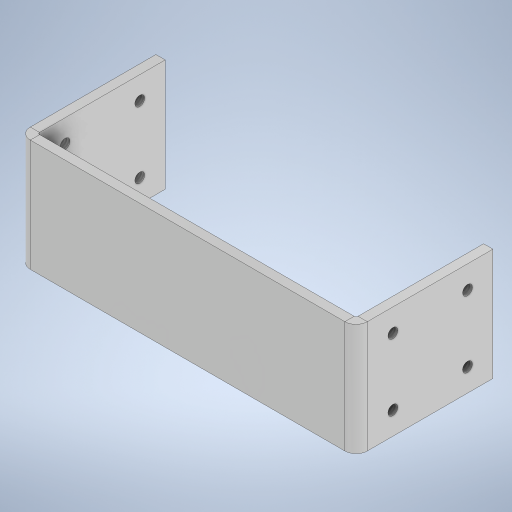
# Autodesk Inventor part: axis_3_bottom_frame(middle)
Saved by Autodesk Inventor 2024.1 (Build 281209000, 209)
## iProperties
Created: 2023-09-23
Part Number: axis_3_bottom_frame(middle)
Material: Aluminum 6061-AHC
Document SubType Name: Sheet Metal
Designer: chanh
Density: 2.7 g/cm^3
Sheet Metal Rule: Default_mm
Appearance: Aluminum - Dark
Author: chanh
Autodesk Inventor part; units mm, degrees
ref_plane "YZ Plane" through (0, 0, 0) normal (1, 0, 0) x (0, 1, 0)
ref_plane "XZ Plane" through (0, 0, 0) normal (0, 1, 0) x (-1, 0, 0)
ref_plane "XY Plane" through (0, 0, 0) normal (0, 0, 1) x (1, 0, 0)
sketch "Sketch1" plane through (0, 0, 0) normal (0, 0, 1) x (1, 0, 0)
  line L0 (27.09, -9) -> (-27.09, -9)
  line L1 (-27.09, -9) -> (-27.09, 9)
  line L2 (-27.09, 9) -> (27.09, 9)
  line L3 (27.09, 9) -> (27.09, -9)
  line L4 (27.09, -9) -> (-27.09, 9) construction
  line L5 (-27.09, -9) -> (27.09, 9) construction
  point P0 (0, 0)
  dimension "d0" = 54.18
  dimension "d1" = 18
  measures "d0" distance of L1.end L2.end
  measures "d1" distance of L0.end L1.end
extrude "Plate1" add sketch "Sketch1" along normal blind 1.5
sketch "Sketch2" plane through (-25.59, 9, 1.5) normal (-1, 0, 0) x (0, -1, 0)
  line L0 (18, 0) -> (0, 0)
  line L1 (0, 0) -> (0, -22)
  line L2 (0, -22) -> (18, -22)
  line L3 (18, -22) -> (18, 0)
  constraints: 6 end point, 1 horizontal, 1 perpendicular, 1 vertical
edge flange "Flange1" height 22 angle 90 thickness 1.5 bend radius 0.31 thickness toward (-1, 0, 0) relief straight relief width 1.5 relief depth 0.75 corner gap 0.31 corner form 0 edges at (-27.09, 0, 0) (27.09, 0, 0) wall of the first edge with corners at (-25.59, -9, 1.5) (-25.59, 9, 1.5) (-25.59, 9, -20.5) (-25.59, -9, -20.5)
bend "Bend1"
corner "Corner1"
sketch "Sketch3" plane through (27.09, -9, -20.5) normal (1, 0, 0) x (0, 0, -1)
  line L0 (-20.19, 18) -> (-20.19, 0) construction
  line L1 (0, 0) -> (-20.19, 0) construction
  line L2 (0, 18) -> (0, 0) construction
  line L3 (-20.19, 18) -> (0, 18) construction
  line L4 (0, 18) -> (-20.19, 0) construction
  line L5 (0, 0) -> (-20.19, 18) construction
  point P0 (-20.5, 9)
  point P1 (-16.095, 14.3492)
  point P2 (-4.095, 14.3492)
  point P3 (-16.095, 3.6508)
  point P4 (-4.095, 3.6508)
  dimension "d13" = 12
  constraints: 4 end point, 4 point on line, 2 horizontal alignment, 1 vertical alignment
  measures "d13" distance of point (-4.095, 14.349) point (-16.095, 14.349)
hole "Hole1" at (27.09, 5.3492, -4.405) at (27.09, 5.3492, -16.405) at (27.09, -5.3492, -4.405) at (27.09, -5.3492, -16.405) direction (-1, 0, 0) diameter 1.567 end through all thread size "M2x0.4" class "6H" standard "ISO Metric profile"
equation "\"d2\" = Thickness"
equation "\"d3\" = BendReliefWidth"
equation "\"d4\" = BendReliefDepth"
equation "\"d5\" = MinimumRemnant"
equation "\"d6\" = TransitionRadius"
equation "\"d9\" = BendRadius"
equation "\"d10\" = CornerReliefSize"
equation "\"d11\" = GapSize"
equation "\"d12\" = JacobiRadiusSize"
equation "\"BendReliefWidth\" = Thickness"
equation "\"BendReliefDepth\" = 0.5 * Thickness"
equation "\"CornerReliefSize\" = 4 * Thickness"
equation "\"MinimumRemnant\" = 2 * Thickness"
equation "\"TransitionRadius\" = BendRadius"
equation "\"JacobiRadiusSize\" = BendRadius"
equation "\"GapSize\" = Thickness"
equation "\"Thickness\" = 1.5"
equation "\"BendRadius\" = 0.31"
body "Solid1"
